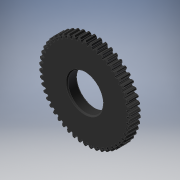
# Autodesk Inventor part: GEFHBS0.5-50-3-10-W0_b
Saved by Autodesk Inventor 2019 (Build 230136000, 136)
## iProperties
Created: 2022-10-16
Part Number: GEFHBS0.5-50-3-10-W0_b
Material: Generic
Catalog Web Link: www.cadenas.de
Description: GEFHB, GEFHBB, GEFHBG, GEFHBS, GEFB, GEFBB, GEFBG, GEFBS, GEFKB, GEFKBB, GEFKBG, GEFKBS_body-Spur Gears - Tooth Width, Hub Dimensions Configurable - Pressure Angle 20degree Module 0.5 / 0.8 / 1.0 / 1.5 / 2.0 / 2.5 / 3.0
Vendor: MISUMI
Document SubType Name: Modeling
Designer: psAdmin
Manufacturer: MISUMI
Mass: 1.22085 g
Surface Area: 13.5083 cm^2
Volume: 1.22085 cm^3
Density: 1 g/cm^3
Appearance: PSOLRGB-175-175-175
Category: PARTsolutions
Company: MISUMI
Title: GEFHBS0.5-50-3-10-W0
Author: Cadenas PARTsolutions
Comments: Spur Gears - Tooth Width, Hub Dimensions Configurable - Pressure Angle 20degree Module 0.5 / 0.8 / 1.0 / 1.5 / 2.0 / 2.5 / 3.0
PSOL_IDENT_0: {$CADENAS_DATA/23d-libs/misumi/metric/54_spur_gears/gefhb/gefhb.prj},485 {VTYP=3D},{NB=GEFHBS0.5-50-
PSOL_IDENT_1: 3-10-W0_b},{LINA=GEFHBS0.5-50-3-10-W0},{NN=GEFHB, GEFHBB, GEFHBG, GEFHBS, GEFB, GEFBB, GEFBG, GEFBS,
PSOL_IDENT_2: GEFKB, GEFKBB, GEFKBG, GEFKBS_body},{DATE=07.06.2021 01:25:58},{GEOMDATE=09.07.2020 06:30:05},{VERS
PSOL_IDENT_3: ION=},{LINEID=10},{WBVAR=SHS,MAT,ST,NT,B,PS,ALT2,TPC,W,H,ALT1,ALT11,ALT4,Z,J,ALT5,Q,R,S,T,ALT9,SRG,A
PSOL_IDENT_4: LT6,LFC,LTC,MALT6,ALT7,KFC,KTC,K,ALT3,DIRALT3,QFC,QTC,MALT3,ALT8,DIRALT8,ZFC,ZTC,U},{WBNUMERIC=NT,B,
PSOL_IDENT_5: W,H,Z,J,Q,R,S,T,SRG,LFC,LTC,KFC,KTC,K,QFC,QTC,ZFC,ZTC,U}  {NB=GEFHBS0.5-50-3-10-W0_b},{LINA=GEFHBS0.
PSOL_IDENT_6: 5-50-3-10-W0},{KT=DUMMY},{PN=GEFHBS0.5-50-3-10-W0},{TYPE=GEFHBS},{SHS=RH},{SHSALG= 'RH','Round Hole'
PSOL_IDENT_7: ,'RHT','Round Hole+Tap' },{MAT=SUS304},{MATALG='S45C', 'S45C Equivalent', 'SUS304', 'SUS304'},{ST=},
PSOL_IDENT_8: {STALG= '','-'},{MOD=0.5},{MOD1=0.5},{AC=N/A},{NT=50},{NTALG=20,24,25,26,30,32,36,40,48,50},{NTALG1=
PSOL_IDENT_9: 20,24,25,26,30,32,36,40,48,50},{NTALG2=0},{NTALG3=24,25,26,30,32,36,40,48,50},{B=3},{BA=[2:5/1]},{PS=
PSOL_IDENT_10: 10},{PALG='3','3','4','4','5','5','6','6','6.35','6.35','7','7','8','8','9','9','10','10','11','11','
PSOL_IDENT_11: 12','12'},{PA1='3','3','4','4','5','5','6','6','6.35','6.35','7','7','8','8','9','9','10','10','11','
PSOL_IDENT_12: 11','12','12'},{PA2='0'},{PA3='3','3','4','4','5','5','6','6','6.35','6.35','7','7','8','8','9','9','
PSOL_IDENT_13: 10','10','11','11','12','12'},{P=10.00},{P2=10},{ALT2=},{ALT2ALG='','N/A'},{TPC=N/A},{TPCALG= 'N/A'
PSOL_IDENT_14: },{ALT2PN=},{W=0},{WA=[0:10/1]},{WMA=0},{H=0},{HA=0},{HMIN=12.0},{HMAX=21},{HPN=},{DD=25.0},{D=26.0}
PSOL_IDENT_15: ,{G=23.75},{M=-},{ML=0},{ACSS=-},{BB=0},{TT=0.0},{L=3},{LL2=0},{ALT1=},{ALT1ALG= '','N/A' },{ALT1PN=
PSOL_IDENT_16: },{KC=0.000},{ALT11=},{ALT11ALG= '','N/A' },{ALT11PN=},{DEG=0},{ALT4=},{ALT4ALG='','Not applicable'}
PSOL_IDENT_17: ,{ALT4PN=},{ALT41=0},{ALT42=0},{Z=0},{ZMINL=12},{ZMAXL=19},{ZMINR=12},{ZMAXR=19},{ZALG=0},{ZPN=},{J=
PSOL_IDENT_18: 0.0},{JALG=0},{JMIN=2},{JMAX=0},{JPN=},{ALT5=},{ALT5ALG= '','Not applicable' },{ALT5PN=},{Q=0},{QALG=
PSOL_IDENT_19: 0},{QMIN=12},{QMAX=19},{QPN=},{R=0},{RALG=0},{RMIN=12},{RMAX=19},{RPN=},{S=0},{SALG=0},{SMIN=3},{SMA
PSOL_IDENT_20: X=-3},{SPN=},{T=0},{TALG=0},{TMIN=3},{TMAX=0},{TPN=},{ALT9=},{ALT9ALG= '','Not applicable' },{SRG=0.
PSOL_IDENT_21: 0},{SRGALG=0},{SRGMIN=3.500},{SRGMINALG=3.500},{SRGMAX=0.000},{SRGMAXALG=0.000},{DD2=0.0},{MM=0.00},
PSOL_IDENT_22: {NN=0.00},{DD2ALG=0.000},{MMALG=0.000},{NNALG=0.000},{ALT9PN=},{ALT6=},{ALT6ALG= '','Not applicable'
PSOL_IDENT_23: },{ALT6PN=},{LFC=0},{LFCALG=0},{LTC=0},{LTCALG=0},{LPCDMIN=18},{LPCDMAX=16},{MALT6=N/A},{MALT6ALG= '
PSOL_IDENT_24: N/A' },{C=0.0},{ALT7=},{ALT7ALG= '','Not applicable' },{ALT7PN=},{KFC=0},{KFCALG=[0]},{KTC=0},{KTCAL
PSOL_IDENT_25: G=[0]},{KPCDMIN1=17},{KPCDMAX1=-7},{KPCDMIN2=7},{KPCDMAX2=16},{K=0.0},{KALG=[0]},{KALT7L=3},{TIF=1},
PSOL_IDENT_26: {KPCD=0},{SCREW=0},{SCREWL=6},{PLANE=5},{PLANE1=5},{ALT3=},{ALT3ALG= '','Not applicable' },{ALT3PN=}
PSOL_IDENT_27: ,{DIRALT3=},{DIRALT3ALG= '','N/A' },{QFC=0},{QFCALG=[0]},{QTC=0},{QTCALG=[0]},{QPCDMIN1=17},{QPCDMAX
PSOL_IDENT_28: 1=-7},{QPCDMIN2=7},{QPCDMAX2=16},{QPCD=0},{CIFMALT3=3},{MALT3=N/A},{MALT3ALG= 'N/A' },{MALT3L=0},{MS
PSOL_IDENT_29: 1=3},{MMAX=1},{MIN=2},{MAX=2},{PITCH=0},{ALT8=},{ALT8ALG= '','Not applicable' },{ALT8PN=},{DIRALT8=}
PSOL_IDENT_30: ,{DIRALT8ALG= '','N/A' },{ZFC=0},{ZFCALG=[0]},{ZTC=0},{ZTCALG=[0]},{ZPCDMIN1=20},{ZPCDMIN2=11},{ZPCD
PSOL_IDENT_31: MAX1=-10},{ZPCDMAX2=13},{ZPCD=0},{U=0},{UALG=[0]},{UMAX=0},{UMAX1=0},{UMAX2=0},{UMIN=3},{U1=0.0},{U2=
PSOL_IDENT_32: 0.0},{F=0.0},{LL13D=0},{LL23D=0},{PZQRDD2=10},{LBS=3},{PCD=0},{SHN=0},{SHDEG1=0},{SHDEG2=0},{ALT3LBS=
PSOL_IDENT_33: 2.5},{D1=1.8},{D2=3.6},{D3=20},{D4=0.05},{D5=4.166667},{D6=3.846154},{D7=0.425},{D8=0.25},{D9=0.4133
PSOL_IDENT_34: 12},{S1=15},{S2=0.5}
NB: GEFHBS0.5-50-3-10-W0_b
NN: 0
NT: 50
NBSYN: $PN._b
LINA: GEFHBS0.5-50-3-10-W0
CATALOG: Misumi
PN: GEFHBS0.5-50-3-10-W0
SHS: Round Hole
MAT: SUS304
ST: -
MOD: 0.5
B: 3
PS: 10
ALT2: N/A
TPC: N/A
W: 0
H: 0
DD: 25
D: 26
G: 23.75
M: -
ACSS: -
ALT1: N/A
ALT11: N/A
ALT4: Not applicable
Z: 0
J: 0
ALT5: Not applicable
Q: 0
R: 0
S: 0
T: 0
ALT9: Not applicable
SRG: 0
DD2: 0
MM: 0
ALT6: Not applicable
LFC: 0
LTC: 0
MALT6: N/A
C: 0
ALT7: Not applicable
KFC: 0
KTC: 0
K: 0
ALT3: Not applicable
DIRALT3: N/A
QFC: 0
QTC: 0
MALT3: N/A
ALT8: Not applicable
DIRALT8: N/A
ZFC: 0
ZTC: 0
U: 0
U1: 0
U2: 0
F: 0
SUPPLIER: MISUMI
ARTICLENO: GEFHBS0.5-50-3-10-W0_b
BOMINFO: GEFHBS0.5-50-3-10-W0
CREATOR: CADENAS GmbH
Autodesk Inventor part; units mm, degrees
(part 1 of 2)
sketch "_____14" plane through (0, 0, 0) normal (1, 0, 0) x (0, 0, -1)
  line L0 (0, 0) -> (-3, 0)
  line L1 (-3, 0) -> (-3, 12.5)
  line L2 (-3, 12.5) -> (-2.3301, 15)
  line L3 (-2.3301, 15) -> (-0.6699, 15)
  line L4 (-0.6699, 15) -> (0, 12.5)
  line L5 (0, 12.5) -> (0, 0)
  line L6 (0, 0) -> (-3, 0)
  constraints: 14 end point
revolve "Revolution1" add sketch "_____14" angle 360 about axis through (0, 0, 0) along (0, 0, -1)
sketch "Sketch_3" plane through (0, 0, 0) normal (0, 0, 1) x (1, 0, 0)
  circle A0 centre (0, 0) radius 52
  arc A1 (-12.9833, 0.6584) -> (-12.9575, 0.6121) centre (-12.9334, 0.6559) ccw
  arc A2 (-12.9575, 0.6121) -> (-12.4938, 0.3926) centre (-10.9465, 4.2613) ccw
  arc A3 (-12.4938, 0.3926) -> (-12.425, 0.3718) centre (-12.3403, 0.7764) ccw
  arc A4 (-12.0493, 0.2732) -> (-12.425, 0.3718) centre (-13.2129, -3.3927) ccw
  arc A5 (-11.875, 0.0342) -> (-12.0493, 0.2732) centre (-12.1249, 0.0349) ccw
  arc A6 (-11.875, 0.0342) -> (-11.875, -0.0342) centre (0, 0) ccw
  arc A7 (-12.0493, -0.2732) -> (-11.875, -0.0342) centre (-12.1249, -0.0349) ccw
  arc A8 (-12.425, -0.3718) -> (-12.0493, -0.2732) centre (-13.2129, 3.3927) ccw
  arc A9 (-12.425, -0.3718) -> (-12.4938, -0.3926) centre (-12.3403, -0.7764) ccw
  arc A10 (-12.4938, -0.3926) -> (-12.9575, -0.6121) centre (-10.9465, -4.2613) ccw
  arc A11 (-12.9575, -0.6121) -> (-12.9833, -0.6584) centre (-12.9334, -0.6559) ccw
  arc A12 (-12.9833, -0.6584) -> (-12.9635, -0.974) centre (0, 0) ccw
  arc A13 (-12.9635, -0.974) -> (-12.9321, -1.0167) centre (-12.9136, -0.9703) ccw
  arc A14 (-12.9321, -1.0167) -> (-12.4445, -1.1764) centre (-11.3942, 2.8558) ccw
  arc A15 (-12.4445, -1.1764) -> (-12.3736, -1.1884) centre (-12.3403, -0.7764) ccw
  arc A16 (-11.9885, -1.2392) -> (-12.3736, -1.1884) centre (-12.6835, -5.022) ccw
  arc A17 (-11.7856, -1.4544) -> (-11.9885, -1.2392) centre (-12.0337, -1.485) ccw
  arc A18 (-11.7856, -1.4544) -> (-11.777, -1.5222) centre (0, 0) ccw
  arc A19 (-11.9201, -1.7812) -> (-11.777, -1.5222) centre (-12.025, -1.5543) ccw
  arc A20 (-12.2804, -1.9262) -> (-11.9201, -1.7812) centre (-13.534, 1.71) ccw
  arc A21 (-12.2804, -1.9262) -> (-12.3461, -1.9554) centre (-12.1457, -2.3169) ccw
  arc A22 (-12.3461, -1.9554) -> (-12.7786, -2.2313) centre (-10.3261, -5.5997) ccw
  arc A23 (-12.7786, -2.2313) -> (-12.7984, -2.2805) centre (-12.7492, -2.2717) ccw
  arc A24 (-12.7984, -2.2805) -> (-12.7392, -2.5911) centre (0, 0) ccw
  arc A25 (-12.7392, -2.5911) -> (-12.7027, -2.6295) centre (-12.6902, -2.5811) ccw
  arc A26 (-12.7027, -2.6295) -> (-12.199, -2.7268) centre (-11.6623, 1.4052) ccw
  arc A27 (-12.199, -2.7268) -> (-12.1271, -2.7298) centre (-12.1457, -2.3169) ccw
  arc A28 (-11.7387, -2.732) -> (-12.1271, -2.7298) centre (-11.9541, -6.5721) ccw
  arc A29 (-11.5104, -2.9201) -> (-11.7387, -2.732) centre (-11.7527, -2.9816) ccw
  arc A30 (-11.5104, -2.9201) -> (-11.4934, -2.9863) centre (0, 0) ccw
  arc A31 (-11.6028, -3.2611) -> (-11.4934, -2.9863) centre (-11.7353, -3.0491) ccw
  arc A32 (-11.9422, -3.4501) -> (-11.6028, -3.2611) centre (-13.6416, 0.0002) ccw
  arc A33 (-11.9422, -3.4501) -> (-12.0037, -3.4874) centre (-11.7596, -3.8209) ccw
  arc A34 (-12.0037, -3.4874) -> (-12.3982, -3.8153) centre (-9.5428, -6.8497) ccw
  arc A35 (-12.3982, -3.8153) -> (-12.4117, -3.8666) centre (-12.3639, -3.8517) ccw
  arc A36 (-12.4117, -3.8666) -> (-12.314, -4.1673) centre (0, 0) ccw
  arc A37 (-12.314, -4.1673) -> (-12.2729, -4.2009) centre (-12.2666, -4.1513) ccw
  arc A38 (-12.2729, -4.2009) -> (-11.761, -4.2342) centre (-11.7465, -0.0676) ccw
  arc A39 (-11.761, -4.2342) -> (-11.6894, -4.2282) centre (-11.7596, -3.8209) ccw
  arc A40 (-11.3037, -4.1817) -> (-11.6894, -4.2282) centre (-11.0361, -8.0185) ccw
  arc A41 (-11.0536, -4.3397) -> (-11.3037, -4.1817) centre (-11.2863, -4.4311) ccw
  arc A42 (-11.0536, -4.3397) -> (-11.0285, -4.4032) centre (0, 0) ccw
  arc A43 (-11.1026, -4.6896) -> (-11.0285, -4.4032) centre (-11.2607, -4.4959) ccw
  arc A44 (-11.4156, -4.9197) -> (-11.1026, -4.6896) centre (-13.534, -1.7095) ccw
  arc A45 (-11.4156, -4.9197) -> (-11.4719, -4.9643) centre (-11.188, -5.2646) ccw
  arc A46 (-11.4719, -4.9643) -> (-11.8223, -5.3391) centre (-8.6091, -7.9917) ccw
  arc A47 (-11.8223, -5.3391) -> (-11.8292, -5.3917) centre (-11.7837, -5.3709) ccw
  arc A48 (-11.8292, -5.3917) -> (-11.6946, -5.6778) centre (0, 0) ccw
  arc A49 (-11.6946, -5.6778) -> (-11.6496, -5.7059) centre (-11.6496, -5.6559) ccw
  arc A50 (-11.6496, -5.7059) -> (-11.1376, -5.6749) centre (-11.6454, -1.5393) ccw
  arc A51 (-11.1376, -5.6749) -> (-11.0673, -5.6599) centre (-11.1879, -5.2647) ccw
  arc A52 (-10.6905, -5.5654) -> (-11.0673, -5.6599) centre (-9.9441, -9.3385) ccw
  arc A53 (-10.4226, -5.6909) -> (-10.6905, -5.5654) centre (-10.642, -5.8107) ccw
  arc A54 (-10.4226, -5.6909) -> (-10.3896, -5.7507) centre (0, 0) ccw
  arc A55 (-10.4273, -6.0442) -> (-10.3896, -5.7507) centre (-10.6084, -5.8718) ccw
  arc A56 (-10.709, -6.3116) -> (-10.4273, -6.0442) centre (-13.213, -3.3923) ccw
  arc A57 (-10.709, -6.3116) -> (-10.7593, -6.363) centre (-10.4399, -6.6254) ccw
  arc A58 (-10.7593, -6.363) -> (-11.0599, -6.7787) centre (-7.5396, -9.0077) ccw
  arc A59 (-11.0599, -6.7787) -> (-11.0602, -6.8317) centre (-11.0176, -6.8055) ccw
  arc A60 (-11.0602, -6.8317) -> (-10.8907, -7.0987) centre (0, 0) ccw
  arc A61 (-10.8907, -7.0987) -> (-10.8426, -7.121) centre (-10.8488, -7.0714) ccw
  arc A62 (-10.8426, -7.121) -> (-10.3385, -7.026) centre (-11.3606, -2.9867) ccw
  arc A63 (-10.3385, -7.026) -> (-10.2706, -7.0024) centre (-10.4399, -6.6254) ccw
  arc A64 (-9.9087, -6.8614) -> (-10.2706, -7.0024) centre (-8.6953, -10.5111) ccw
  arc A65 (-9.6271, -6.9523) -> (-9.9087, -6.8614) centre (-9.8298, -7.0986) ccw
  arc A66 (-9.6271, -6.9523) -> (-9.587, -7.0076) centre (0, 0) ccw
  arc A67 (-9.5875, -7.3034) -> (-9.587, -7.0076) centre (-9.7888, -7.1551) ccw
  arc A68 (-9.8335, -7.6041) -> (-9.5875, -7.3034) centre (-12.6837, -5.0216) ccw
  arc A69 (-9.8335, -7.6041) -> (-9.8769, -7.6613) centre (-9.5272, -7.8816) ccw
  arc A70 (-9.8769, -7.6613) -> (-10.1231, -8.1114) centre (-6.3511, -9.8817) ccw
  arc A71 (-10.1231, -8.1114) -> (-10.1167, -8.1641) centre (-10.0778, -8.1327) ccw
  arc A72 (-10.1167, -8.1641) -> (-9.9152, -8.4077) centre (0, 0) ccw
  arc A73 (-9.9152, -8.4077) -> (-9.8646, -8.4238) centre (-9.877, -8.3754) ccw
  arc A74 (-9.8646, -8.4238) -> (-9.3764, -8.2664) centre (-10.8967, -4.387) ccw
  arc A75 (-9.3764, -8.2664) -> (-9.312, -8.2344) centre (-9.5272, -7.8816) ccw
  arc A76 (-8.9706, -8.0492) -> (-9.312, -8.2344) centre (-7.3093, -11.5181) ccw
  arc A77 (-8.6799, -8.1041) -> (-8.9706, -8.0492) centre (-8.8626, -8.2747) ccw
  arc A78 (-8.6799, -8.1041) -> (-8.6331, -8.1539) centre (0, 0) ccw
  arc A79 (-8.5966, -8.4475) -> (-8.6331, -8.1539) centre (-8.8148, -8.3255) ccw
  arc A80 (-8.8029, -8.7766) -> (-8.5966, -8.4475) centre (-11.9543, -6.5717) ccw
  arc A81 (-8.8029, -8.7766) -> (-8.8388, -8.8388) centre (-8.4642, -9.0135) ccw
  arc A82 (-8.8388, -8.8388) -> (-9.0266, -9.3162) centre (-5.0626, -10.5997) ccw
  arc A83 (-9.0266, -9.3162) -> (-9.0137, -9.3677) centre (-8.979, -9.3316) ccw
  arc A84 (-9.0137, -9.3677) -> (-8.7832, -9.5841) centre (0, 0) ccw
  arc A85 (-8.7832, -9.5841) -> (-8.7311, -9.5938) centre (-8.7494, -9.5473) ccw
  arc A86 (-8.7311, -9.5938) -> (-8.2664, -9.3764) centre (-10.2609, -5.7181) ccw
  arc A87 (-8.2664, -9.3764) -> (-8.2065, -9.3366) centre (-8.4642, -9.0135) ccw
  arc A88 (-7.891, -9.11) -> (-8.2065, -9.3366) centre (-5.8081, -12.3433) ccw
  arc A89 (-7.5957, -9.128) -> (-7.891, -9.11) centre (-7.7556, -9.3202) ccw
  arc A90 (-7.5957, -9.128) -> (-7.5431, -9.1716) centre (0, 0) ccw
  arc A91 (-7.47, -9.4583) -> (-7.5431, -9.1716) centre (-7.7019, -9.3647) ccw
  arc A92 (-7.6335, -9.8107) -> (-7.47, -9.4583) centre (-11.0364, -8.0181) ccw
  arc A93 (-7.6335, -9.8107) -> (-7.6613, -9.8769) centre (-7.2678, -10.0033) ccw
  arc A94 (-7.6613, -9.8769) -> (-7.7878, -10.3741) centre (-3.6941, -11.1507) ccw
  arc A95 (-7.7878, -10.3741) -> (-7.7685, -10.4235) centre (-7.7387, -10.3834) ccw
  arc A96 (-7.7685, -10.4235) -> (-7.5127, -10.6094) centre (0, 0) ccw
  arc A97 (-7.5127, -10.6094) -> (-7.4598, -10.6124) centre (-7.4838, -10.5686) ccw
  arc A98 (-7.4598, -10.6124) -> (-7.026, -10.3385) centre (-9.4634, -6.9591) ccw
  arc A99 (-7.026, -10.3385) -> (-6.9716, -10.2915) centre (-7.2678, -10.0033) ccw
  arc A100 (-6.687, -10.0272) -> (-6.9716, -10.2915) centre (-4.2153, -12.974) ccw
  arc A101 (-6.3918, -10.008) -> (-6.687, -10.0272) centre (-6.5263, -10.2187) ccw
  arc A102 (-6.3918, -10.008) -> (-6.3341, -10.0447) centre (0, 0) ccw
  arc A103 (-6.2257, -10.3199) -> (-6.3341, -10.0447) centre (-6.4674, -10.2561) ccw
  arc A104 (-6.3437, -10.69) -> (-6.2257, -10.3199) centre (-9.9444, -9.3381) ccw
  arc A105 (-6.3437, -10.69) -> (-6.363, -10.7593) centre (-5.9568, -10.8353) ccw
  arc A106 (-6.363, -10.7593) -> (-6.4262, -11.2684) centre (-2.2675, -11.5257) ccw
  arc A107 (-6.4262, -11.2684) -> (-6.4009, -11.315) centre (-6.3763, -11.2715) ccw
  arc A108 (-6.4009, -11.315) -> (-6.1238, -11.4673) centre (0, 0) ccw
  arc A109 (-6.1238, -11.4673) -> (-6.0709, -11.4637) centre (-6.1002, -11.4232) ccw
  arc A110 (-6.0709, -11.4637) -> (-5.6749, -11.1376) centre (-8.5165, -8.0903) ccw
  arc A111 (-5.6749, -11.1376) -> (-5.6268, -11.0842) centre (-5.9568, -10.8353) ccw
  arc A112 (-5.3775, -10.7862) -> (-5.6268, -11.0842) centre (-2.5559, -13.4) ccw
  arc A113 (-5.087, -10.7302) -> (-5.3775, -10.7862) centre (-5.1941, -10.9561) ccw
  arc A114 (-5.087, -10.7302) -> (-5.0252, -10.7593) centre (0, 0) ccw
  arc A115 (-4.8832, -11.0189) -> (-5.0252, -10.7593) centre (-5.131, -10.9858) ccw
  arc A116 (-4.9539, -11.4008) -> (-4.8832, -11.0189) centre (-8.6956, -10.5108) ccw
  arc A117 (-4.9539, -11.4008) -> (-4.9643, -11.4719) centre (-4.5518, -11.4964) ccw
  arc A118 (-4.9643, -11.4719) -> (-4.9632, -11.9849) centre (-0.805, -11.719) ccw
  arc A119 (-4.9632, -11.9849) -> (-4.9323, -12.028) centre (-4.9133, -11.9817) ccw
  arc A120 (-4.9323, -12.028) -> (-4.6383, -12.1444) centre (0, 0) ccw
  arc A121 (-4.6383, -12.1444) -> (-4.5862, -12.1342) centre (-4.6204, -12.0977) ccw
  arc A122 (-4.5862, -12.1342) -> (-4.2342, -11.761) centre (-7.4354, -9.0939) ccw
  arc A123 (-4.2342, -11.761) -> (-4.1932, -11.702) centre (-4.5518, -11.4964) ccw
  arc A124 (-3.9832, -11.3752) -> (-4.1932, -11.702) centre (-0.8563, -13.6147) ccw
  arc A125 (-3.7021, -11.2832) -> (-3.9832, -11.3752) centre (-3.78, -11.5207) ccw
  arc A126 (-3.7021, -11.2832) -> (-3.6371, -11.3043) centre (0, 0) ccw
  arc A127 (-3.4636, -11.544) -> (-3.6371, -11.3043) centre (-3.7136, -11.5423) ccw
  arc A128 (-3.4859, -11.9318) -> (-3.4636, -11.544) centre (-7.3097, -11.5178) ccw
  arc A129 (-3.4859, -11.9318) -> (-3.4874, -12.0037) centre (-3.075, -11.9763) ccw
  arc A130 (-3.4874, -12.0037) -> (-3.4219, -12.5125) centre (0.6701, -11.7275) ccw
  arc A131 (-3.4219, -12.5125) -> (-3.3859, -12.5513) centre (-3.3728, -12.5031) ccw
  arc A132 (-3.3859, -12.5513) -> (-3.0796, -12.63) centre (0, 0) ccw
  arc A133 (-3.0796, -12.63) -> (-3.0293, -12.6133) centre (-3.0678, -12.5814) ccw
  arc A134 (-3.0293, -12.6133) -> (-2.7268, -12.199) centre (-6.237, -9.9541) ccw
  arc A135 (-2.7268, -12.199) -> (-2.6935, -12.1353) centre (-3.075, -11.9763) ccw
  arc A136 (-2.5261, -11.7847) -> (-2.6935, -12.1353) centre (0.8568, -13.6146) ccw
  arc A137 (-2.2587, -11.6582) -> (-2.5261, -11.7847) centre (-2.3063, -11.9036) ccw
  arc A138 (-2.2587, -11.6582) -> (-2.1916, -11.671) centre (0, 0) ccw
  arc A139 (-1.9895, -11.8871) -> (-2.1916, -11.671) centre (-2.2377, -11.9167) ccw
  arc A140 (-1.963, -12.2746) -> (-1.9895, -11.8871) centre (-5.8085, -12.3431) ccw
  arc A141 (-1.963, -12.2746) -> (-1.9554, -12.3461) centre (-1.5497, -12.2672) ccw
  arc A142 (-1.9554, -12.3461) -> (-1.8267, -12.8427) centre (2.1347, -11.5511) ccw
  arc A143 (-1.8267, -12.8427) -> (-1.7861, -12.8767) centre (-1.7792, -12.8272) ccw
  arc A144 (-1.7861, -12.8767) -> (-1.4724, -12.9164) centre (0, 0) ccw
  arc A145 (-1.4724, -12.9164) -> (-1.4245, -12.8935) centre (-1.4667, -12.8667) ccw
  arc A146 (-1.4245, -12.8935) -> (-1.1764, -12.4445) centre (-4.9403, -10.6573) ccw
  arc A147 (-1.1764, -12.4445) -> (-1.1513, -12.3771) centre (-1.5497, -12.2672) ccw
  arc A148 (-1.0292, -12.0084) -> (-1.1513, -12.3771) centre (2.5564, -13.3999) ccw
  arc A149 (-0.7797, -11.8494) -> (-1.0292, -12.0084) centre (-0.7961, -12.0988) ccw
  arc A150 (-0.7797, -11.8494) -> (-0.7115, -11.8537) centre (0, 0) ccw
  arc A151 (-0.484, -12.0427) -> (-0.7115, -11.8537) centre (-0.7265, -12.1032) ccw
  arc A152 (-0.4091, -12.4238) -> (-0.484, -12.0427) centre (-4.2157, -12.9738) ccw
  arc A153 (-0.4091, -12.4238) -> (-0.3926, -12.4938) centre (0, -12.3647) ccw
  arc A154 (-0.3926, -12.4938) -> (-0.2027, -12.9704) centre (3.5656, -11.1924) ccw
  arc A155 (-0.2027, -12.9704) -> (-0.1581, -12.999) centre (-0.1575, -12.949) ccw
  arc A156 (-0.1581, -12.999) -> (0.1581, -12.999) centre (0, 0) ccw
  arc A157 (0.1581, -12.999) -> (0.2027, -12.9704) centre (0.1575, -12.949) ccw
  arc A158 (0.2027, -12.9704) -> (0.3926, -12.4938) centre (-3.5656, -11.1924) ccw
  arc A159 (0.3926, -12.4938) -> (0.4091, -12.4238) centre (0, -12.3647) ccw
  arc A160 (0.484, -12.0427) -> (0.4091, -12.4238) centre (4.2157, -12.9738) ccw
  arc A161 (0.7115, -11.8537) -> (0.484, -12.0427) centre (0.7265, -12.1032) ccw
  arc A162 (0.7115, -11.8537) -> (0.7797, -11.8494) centre (0, 0) ccw
  arc A163 (1.0292, -12.0084) -> (0.7797, -11.8494) centre (0.7961, -12.0988) ccw
  arc A164 (1.1513, -12.3771) -> (1.0292, -12.0084) centre (-2.5564, -13.3999) ccw
  arc A165 (1.1513, -12.3771) -> (1.1764, -12.4445) centre (1.5497, -12.2672) ccw
  arc A166 (1.1764, -12.4445) -> (1.4245, -12.8935) centre (4.9403, -10.6573) ccw
  arc A167 (1.4245, -12.8935) -> (1.4724, -12.9164) centre (1.4667, -12.8667) ccw
  arc A168 (1.4724, -12.9164) -> (1.7861, -12.8767) centre (0, 0) ccw
  arc A169 (1.7861, -12.8767) -> (1.8267, -12.8427) centre (1.7792, -12.8272) ccw
  arc A170 (1.8267, -12.8427) -> (1.9554, -12.3461) centre (-2.1347, -11.5511) ccw
  arc A171 (1.9554, -12.3461) -> (1.963, -12.2746) centre (1.5497, -12.2672) ccw
  arc A172 (1.9895, -11.8871) -> (1.963, -12.2746) centre (5.8085, -12.3431) ccw
  arc A173 (2.1916, -11.671) -> (1.9895, -11.8871) centre (2.2377, -11.9167) ccw
  arc A174 (2.1916, -11.671) -> (2.2587, -11.6582) centre (0, 0) ccw
  arc A175 (2.5261, -11.7847) -> (2.2587, -11.6582) centre (2.3063, -11.9036) ccw
  arc A176 (2.6935, -12.1353) -> (2.5261, -11.7847) centre (-0.8568, -13.6146) ccw
  arc A177 (2.6935, -12.1353) -> (2.7268, -12.199) centre (3.075, -11.9763) ccw
  arc A178 (2.7268, -12.199) -> (3.0293, -12.6133) centre (6.237, -9.9541) ccw
  arc A179 (3.0293, -12.6133) -> (3.0796, -12.63) centre (3.0678, -12.5814) ccw
  arc A180 (3.0796, -12.63) -> (3.3859, -12.5513) centre (0, 0) ccw
  arc A181 (3.3859, -12.5513) -> (3.4219, -12.5125) centre (3.3728, -12.5031) ccw
  arc A182 (3.4219, -12.5125) -> (3.4874, -12.0037) centre (-0.6701, -11.7275) ccw
  arc A183 (3.4874, -12.0037) -> (3.4859, -11.9318) centre (3.075, -11.9763) ccw
  arc A184 (3.4636, -11.544) -> (3.4859, -11.9318) centre (7.3097, -11.5178) ccw
  arc A185 (3.6371, -11.3043) -> (3.4636, -11.544) centre (3.7136, -11.5423) ccw
  arc A186 (3.6371, -11.3043) -> (3.7021, -11.2832) centre (0, 0) ccw
  arc A187 (3.9832, -11.3752) -> (3.7021, -11.2832) centre (3.78, -11.5207) ccw
  arc A188 (4.1932, -11.702) -> (3.9832, -11.3752) centre (0.8563, -13.6147) ccw
  arc A189 (4.1932, -11.702) -> (4.2342, -11.761) centre (4.5518, -11.4964) ccw
  arc A190 (4.2342, -11.761) -> (4.5862, -12.1342) centre (7.4354, -9.0939) ccw
  arc A191 (4.5862, -12.1342) -> (4.6383, -12.1444) centre (4.6204, -12.0977) ccw
  arc A192 (4.6383, -12.1444) -> (4.9323, -12.028) centre (0, 0) ccw
  arc A193 (4.9323, -12.028) -> (4.9632, -11.9849) centre (4.9133, -11.9817) ccw
  arc A194 (4.9632, -11.9849) -> (4.9643, -11.4719) centre (0.805, -11.719) ccw
  arc A195 (4.9643, -11.4719) -> (4.9539, -11.4008) centre (4.5518, -11.4964) ccw
  arc A196 (4.8832, -11.0189) -> (4.9539, -11.4008) centre (8.6956, -10.5108) ccw
  arc A197 (5.0252, -10.7593) -> (4.8832, -11.0189) centre (5.131, -10.9858) ccw
  arc A198 (5.0252, -10.7593) -> (5.087, -10.7302) centre (0, 0) ccw
  arc A199 (5.3775, -10.7862) -> (5.087, -10.7302) centre (5.1941, -10.9561) ccw
  arc A200 (5.6268, -11.0842) -> (5.3775, -10.7862) centre (2.5559, -13.4) ccw
  arc A201 (5.6268, -11.0842) -> (5.6749, -11.1376) centre (5.9568, -10.8353) ccw
  arc A202 (5.6749, -11.1376) -> (6.0709, -11.4637) centre (8.5165, -8.0903) ccw
  arc A203 (6.0709, -11.4637) -> (6.1238, -11.4673) centre (6.1002, -11.4232) ccw
  arc A204 (6.1238, -11.4673) -> (6.4009, -11.315) centre (0, 0) ccw
  arc A205 (6.4009, -11.315) -> (6.4262, -11.2684) centre (6.3763, -11.2715) ccw
  arc A206 (6.4262, -11.2684) -> (6.363, -10.7593) centre (2.2675, -11.5257) ccw
  arc A207 (6.363, -10.7593) -> (6.3437, -10.69) centre (5.9568, -10.8353) ccw
  arc A208 (6.2257, -10.3199) -> (6.3437, -10.69) centre (9.9444, -9.3381) ccw
  arc A209 (6.3341, -10.0447) -> (6.2257, -10.3199) centre (6.4674, -10.2561) ccw
  arc A210 (6.3341, -10.0447) -> (6.3918, -10.008) centre (0, 0) ccw
  arc A211 (6.687, -10.0272) -> (6.3918, -10.008) centre (6.5263, -10.2187) ccw
  arc A212 (6.9716, -10.2915) -> (6.687, -10.0272) centre (4.2153, -12.974) ccw
  arc A213 (6.9716, -10.2915) -> (7.026, -10.3385) centre (7.2678, -10.0033) ccw
  arc A214 (7.026, -10.3385) -> (7.4598, -10.6124) centre (9.4634, -6.9591) ccw
  arc A215 (7.4598, -10.6124) -> (7.5127, -10.6094) centre (7.4838, -10.5686) ccw
  arc A216 (7.5127, -10.6094) -> (7.7685, -10.4235) centre (0, 0) ccw
  arc A217 (7.7685, -10.4235) -> (7.7878, -10.3741) centre (7.7387, -10.3834) ccw
  arc A218 (7.7878, -10.3741) -> (7.6613, -9.8769) centre (3.6941, -11.1507) ccw
  arc A219 (7.6613, -9.8769) -> (7.6335, -9.8107) centre (7.2678, -10.0033) ccw
  arc A220 (7.47, -9.4583) -> (7.6335, -9.8107) centre (11.0364, -8.0181) ccw
  arc A221 (7.5431, -9.1716) -> (7.47, -9.4583) centre (7.7019, -9.3647) ccw
  arc A222 (7.5431, -9.1716) -> (7.5957, -9.128) centre (0, 0) ccw
  arc A223 (7.891, -9.11) -> (7.5957, -9.128) centre (7.7556, -9.3202) ccw
  arc A224 (8.2065, -9.3366) -> (7.891, -9.11) centre (5.8081, -12.3433) ccw
  arc A225 (8.2065, -9.3366) -> (8.2664, -9.3764) centre (8.4642, -9.0135) ccw
  arc A226 (8.2664, -9.3764) -> (8.7311, -9.5938) centre (10.2609, -5.7181) ccw
  arc A227 (8.7311, -9.5938) -> (8.7832, -9.5841) centre (8.7494, -9.5473) ccw
  arc A228 (8.7832, -9.5841) -> (9.0137, -9.3677) centre (0, 0) ccw
  arc A229 (9.0137, -9.3677) -> (9.0266, -9.3162) centre (8.979, -9.3316) ccw
  arc A230 (9.0266, -9.3162) -> (8.8388, -8.8388) centre (5.0626, -10.5997) ccw
  arc A231 (8.8388, -8.8388) -> (8.8029, -8.7766) centre (8.4642, -9.0135) ccw
  arc A232 (8.5966, -8.4475) -> (8.8029, -8.7766) centre (11.9543, -6.5717) ccw
  arc A233 (8.6331, -8.1539) -> (8.5966, -8.4475) centre (8.8148, -8.3255) ccw
  arc A234 (8.6331, -8.1539) -> (8.6799, -8.1041) centre (0, 0) ccw
  arc A235 (8.9706, -8.0492) -> (8.6799, -8.1041) centre (8.8626, -8.2747) ccw
  arc A236 (9.312, -8.2344) -> (8.9706, -8.0492) centre (7.3093, -11.5181) ccw
  arc A237 (9.312, -8.2344) -> (9.3764, -8.2664) centre (9.5272, -7.8816) ccw
  arc A238 (9.3764, -8.2664) -> (9.8646, -8.4238) centre (10.8967, -4.387) ccw
  arc A239 (9.8646, -8.4238) -> (9.9152, -8.4077) centre (9.877, -8.3754) ccw
  arc A240 (9.9152, -8.4077) -> (10.1167, -8.1641) centre (0, 0) ccw
  arc A241 (10.1167, -8.1641) -> (10.1231, -8.1114) centre (10.0778, -8.1327) ccw
  arc A242 (10.1231, -8.1114) -> (9.8769, -7.6613) centre (6.3511, -9.8817) ccw
  arc A243 (9.8769, -7.6613) -> (9.8335, -7.6041) centre (9.5272, -7.8816) ccw
  arc A244 (9.5875, -7.3034) -> (9.8335, -7.6041) centre (12.6837, -5.0216) ccw
  arc A245 (9.587, -7.0076) -> (9.5875, -7.3034) centre (9.7888, -7.1551) ccw
  arc A246 (9.587, -7.0076) -> (9.6271, -6.9523) centre (0, 0) ccw
  arc A247 (9.9087, -6.8614) -> (9.6271, -6.9523) centre (9.8298, -7.0986) ccw
  arc A248 (10.2706, -7.0024) -> (9.9087, -6.8614) centre (8.6953, -10.5111) ccw
  arc A249 (10.2706, -7.0024) -> (10.3385, -7.026) centre (10.4399, -6.6254) ccw
  arc A250 (10.3385, -7.026) -> (10.8426, -7.121) centre (11.3606, -2.9867) ccw
  arc A251 (10.8426, -7.121) -> (10.8907, -7.0987) centre (10.8488, -7.0714) ccw
  arc A252 (10.8907, -7.0987) -> (11.0602, -6.8317) centre (0, 0) ccw
  arc A253 (11.0602, -6.8317) -> (11.0599, -6.7787) centre (11.0176, -6.8055) ccw
  arc A254 (11.0599, -6.7787) -> (10.7593, -6.363) centre (7.5396, -9.0077) ccw
  arc A255 (10.7593, -6.363) -> (10.709, -6.3116) centre (10.4399, -6.6254) ccw
  arc A256 (10.4273, -6.0442) -> (10.709, -6.3116) centre (13.213, -3.3923) ccw
  arc A257 (10.3896, -5.7507) -> (10.4273, -6.0442) centre (10.6084, -5.8718) ccw
  arc A258 (10.3896, -5.7507) -> (10.4226, -5.6909) centre (0, 0) ccw
  arc A259 (10.6905, -5.5654) -> (10.4226, -5.6909) centre (10.642, -5.8107) ccw
  arc A260 (11.0673, -5.6599) -> (10.6905, -5.5654) centre (9.9441, -9.3385) ccw
  arc A261 (11.0673, -5.6599) -> (11.1376, -5.6749) centre (11.1879, -5.2647) ccw
  arc A262 (11.1376, -5.6749) -> (11.6496, -5.7059) centre (11.6454, -1.5393) ccw
  arc A263 (11.6496, -5.7059) -> (11.6946, -5.6778) centre (11.6496, -5.6559) ccw
  arc A264 (11.6946, -5.6778) -> (11.8292, -5.3917) centre (0, 0) ccw
  arc A265 (11.8292, -5.3917) -> (11.8223, -5.3391) centre (11.7837, -5.3709) ccw
  arc A266 (11.8223, -5.3391) -> (11.4719, -4.9643) centre (8.6091, -7.9917) ccw
  arc A267 (11.4719, -4.9643) -> (11.4156, -4.9197) centre (11.188, -5.2646) ccw
  arc A268 (11.1026, -4.6896) -> (11.4156, -4.9197) centre (13.534, -1.7095) ccw
  arc A269 (11.0285, -4.4032) -> (11.1026, -4.6896) centre (11.2607, -4.4959) ccw
  arc A270 (11.0285, -4.4032) -> (11.0536, -4.3397) centre (0, 0) ccw
  arc A271 (11.3037, -4.1817) -> (11.0536, -4.3397) centre (11.2863, -4.4311) ccw
  arc A272 (11.6894, -4.2282) -> (11.3037, -4.1817) centre (11.0361, -8.0185) ccw
  arc A273 (11.6894, -4.2282) -> (11.761, -4.2342) centre (11.7596, -3.8209) ccw
  arc A274 (11.761, -4.2342) -> (12.2729, -4.2009) centre (11.7465, -0.0676) ccw
  arc A275 (12.2729, -4.2009) -> (12.314, -4.1673) centre (12.2666, -4.1513) ccw
  arc A276 (12.314, -4.1673) -> (12.4117, -3.8666) centre (0, 0) ccw
  arc A277 (12.4117, -3.8666) -> (12.3982, -3.8153) centre (12.3639, -3.8517) ccw
  arc A278 (12.3982, -3.8153) -> (12.0037, -3.4874) centre (9.5428, -6.8497) ccw
  arc A279 (12.0037, -3.4874) -> (11.9422, -3.4501) centre (11.7596, -3.8209) ccw
  arc A280 (11.6028, -3.2611) -> (11.9422, -3.4501) centre (13.6416, 0.0002) ccw
  arc A281 (11.4934, -2.9863) -> (11.6028, -3.2611) centre (11.7353, -3.0491) ccw
  arc A282 (11.4934, -2.9863) -> (11.5104, -2.9201) centre (0, 0) ccw
  arc A283 (11.7387, -2.732) -> (11.5104, -2.9201) centre (11.7527, -2.9816) ccw
  arc A284 (12.1271, -2.7298) -> (11.7387, -2.732) centre (11.9541, -6.5721) ccw
  arc A285 (12.1271, -2.7298) -> (12.199, -2.7268) centre (12.1457, -2.3169) ccw
  arc A286 (12.199, -2.7268) -> (12.7027, -2.6295) centre (11.6623, 1.4052) ccw
  arc A287 (12.7027, -2.6295) -> (12.7392, -2.5911) centre (12.6902, -2.5811) ccw
  arc A288 (12.7392, -2.5911) -> (12.7984, -2.2805) centre (0, 0) ccw
  arc A289 (12.7984, -2.2805) -> (12.7786, -2.2313) centre (12.7492, -2.2717) ccw
  arc A290 (12.7786, -2.2313) -> (12.3461, -1.9554) centre (10.3261, -5.5997) ccw
  arc A291 (12.3461, -1.9554) -> (12.2804, -1.9262) centre (12.1457, -2.3169) ccw
  arc A292 (11.9201, -1.7812) -> (12.2804, -1.9262) centre (13.534, 1.71) ccw
  arc A293 (11.777, -1.5222) -> (11.9201, -1.7812) centre (12.025, -1.5543) ccw
  arc A294 (11.777, -1.5222) -> (11.7856, -1.4544) centre (0, 0) ccw
  arc A295 (11.9885, -1.2392) -> (11.7856, -1.4544) centre (12.0337, -1.485) ccw
  arc A296 (12.3736, -1.1884) -> (11.9885, -1.2392) centre (12.6835, -5.022) ccw
  arc A297 (12.3736, -1.1884) -> (12.4445, -1.1764) centre (12.3403, -0.7764) ccw
  arc A298 (12.4445, -1.1764) -> (12.9321, -1.0167) centre (11.3942, 2.8558) ccw
  arc A299 (12.9321, -1.0167) -> (12.9635, -0.974) centre (12.9136, -0.9703) ccw
  arc A300 (12.9635, -0.974) -> (12.9833, -0.6584) centre (0, 0) ccw
  arc A301 (12.9833, -0.6584) -> (12.9575, -0.6121) centre (12.9334, -0.6559) ccw
  arc A302 (12.9575, -0.6121) -> (12.4938, -0.3926) centre (10.9465, -4.2613) ccw
  arc A303 (12.4938, -0.3926) -> (12.425, -0.3718) centre (12.3403, -0.7764) ccw
  arc A304 (12.0493, -0.2732) -> (12.425, -0.3718) centre (13.2129, 3.3927) ccw
  arc A305 (11.875, -0.0342) -> (12.0493, -0.2732) centre (12.1249, -0.0349) ccw
  arc A306 (11.875, -0.0342) -> (11.875, 0.0342) centre (0, 0) ccw
  arc A307 (12.0493, 0.2732) -> (11.875, 0.0342) centre (12.1249, 0.0349) ccw
  arc A308 (12.425, 0.3718) -> (12.0493, 0.2732) centre (13.2129, -3.3927) ccw
  arc A309 (12.425, 0.3718) -> (12.4938, 0.3926) centre (12.3403, 0.7764) ccw
  arc A310 (12.4938, 0.3926) -> (12.9575, 0.6121) centre (10.9465, 4.2613) ccw
  arc A311 (12.9575, 0.6121) -> (12.9833, 0.6584) centre (12.9334, 0.6559) ccw
  arc A312 (12.9833, 0.6584) -> (12.9635, 0.974) centre (0, 0) ccw
  arc A313 (12.9635, 0.974) -> (12.9321, 1.0167) centre (12.9136, 0.9703) ccw
  arc A314 (12.9321, 1.0167) -> (12.4445, 1.1764) centre (11.3942, -2.8558) ccw
  arc A315 (12.4445, 1.1764) -> (12.3736, 1.1884) centre (12.3403, 0.7764) ccw
  arc A316 (11.9885, 1.2392) -> (12.3736, 1.1884) centre (12.6835, 5.022) ccw
  arc A317 (11.7856, 1.4544) -> (11.9885, 1.2392) centre (12.0337, 1.485) ccw
  arc A318 (11.7856, 1.4544) -> (11.777, 1.5222) centre (0, 0) ccw
  arc A319 (11.9201, 1.7812) -> (11.777, 1.5222) centre (12.025, 1.5543) ccw
  arc A320 (12.2804, 1.9262) -> (11.9201, 1.7812) centre (13.534, -1.71) ccw
  arc A321 (12.2804, 1.9262) -> (12.3461, 1.9554) centre (12.1457, 2.3169) ccw
  arc A322 (12.3461, 1.9554) -> (12.7786, 2.2313) centre (10.3261, 5.5997) ccw
  arc A323 (12.7786, 2.2313) -> (12.7984, 2.2805) centre (12.7492, 2.2717) ccw
  arc A324 (12.7984, 2.2805) -> (12.7392, 2.5911) centre (0, 0) ccw
  arc A325 (12.7392, 2.5911) -> (12.7027, 2.6295) centre (12.6902, 2.5811) ccw
  arc A326 (12.7027, 2.6295) -> (12.199, 2.7268) centre (11.6623, -1.4052) ccw
  arc A327 (12.199, 2.7268) -> (12.1271, 2.7298) centre (12.1457, 2.3169) ccw
  arc A328 (11.7387, 2.732) -> (12.1271, 2.7298) centre (11.9541, 6.5721) ccw
  arc A329 (11.5104, 2.9201) -> (11.7387, 2.732) centre (11.7527, 2.9816) ccw
  arc A330 (11.5104, 2.9201) -> (11.4934, 2.9863) centre (0, 0) ccw
  arc A331 (11.6028, 3.2611) -> (11.4934, 2.9863) centre (11.7353, 3.0491) ccw
  arc A332 (11.9422, 3.4501) -> (11.6028, 3.2611) centre (13.6416, -0.0002) ccw
  arc A333 (11.9422, 3.4501) -> (12.0037, 3.4874) centre (11.7596, 3.8209) ccw
  arc A334 (12.0037, 3.4874) -> (12.3982, 3.8153) centre (9.5428, 6.8497) ccw
  arc A335 (12.3982, 3.8153) -> (12.4117, 3.8666) centre (12.3639, 3.8517) ccw
  arc A336 (12.4117, 3.8666) -> (12.314, 4.1673) centre (0, 0) ccw
  arc A337 (12.314, 4.1673) -> (12.2729, 4.2009) centre (12.2666, 4.1513) ccw
  arc A338 (12.2729, 4.2009) -> (11.761, 4.2342) centre (11.7465, 0.0676) ccw
  arc A339 (11.761, 4.2342) -> (11.6894, 4.2282) centre (11.7596, 3.8209) ccw
  arc A340 (11.3037, 4.1817) -> (11.6894, 4.2282) centre (11.0361, 8.0185) ccw
  arc A341 (11.0536, 4.3397) -> (11.3037, 4.1817) centre (11.2863, 4.4311) ccw
  arc A342 (11.0536, 4.3397) -> (11.0285, 4.4032) centre (0, 0) ccw
  arc A343 (11.1026, 4.6896) -> (11.0285, 4.4032) centre (11.2607, 4.4959) ccw
  arc A344 (11.4156, 4.9197) -> (11.1026, 4.6896) centre (13.534, 1.7095) ccw
  arc A345 (11.4156, 4.9197) -> (11.4719, 4.9643) centre (11.188, 5.2646) ccw
  arc A346 (11.4719, 4.9643) -> (11.8223, 5.3391) centre (8.6091, 7.9917) ccw
  arc A347 (11.8223, 5.3391) -> (11.8292, 5.3917) centre (11.7837, 5.3709) ccw
  arc A348 (11.8292, 5.3917) -> (11.6946, 5.6778) centre (0, 0) ccw
  arc A349 (11.6946, 5.6778) -> (11.6496, 5.7059) centre (11.6496, 5.6559) ccw
  arc A350 (11.6496, 5.7059) -> (11.1376, 5.6749) centre (11.6454, 1.5393) ccw
  arc A351 (11.1376, 5.6749) -> (11.0673, 5.6599) centre (11.1879, 5.2647) ccw
  arc A352 (10.6905, 5.5654) -> (11.0673, 5.6599) centre (9.9441, 9.3385) ccw
  arc A353 (10.4226, 5.6909) -> (10.6905, 5.5654) centre (10.642, 5.8107) ccw
  arc A354 (10.4226, 5.6909) -> (10.3896, 5.7507) centre (0, 0) ccw
  arc A355 (10.4273, 6.0442) -> (10.3896, 5.7507) centre (10.6084, 5.8718) ccw
  arc A356 (10.709, 6.3116) -> (10.4273, 6.0442) centre (13.213, 3.3923) ccw
  arc A357 (10.709, 6.3116) -> (10.7593, 6.363) centre (10.4399, 6.6254) ccw
  arc A358 (10.7593, 6.363) -> (11.0599, 6.7787) centre (7.5396, 9.0077) ccw
  arc A359 (11.0599, 6.7787) -> (11.0602, 6.8317) centre (11.0176, 6.8055) ccw
  arc A360 (11.0602, 6.8317) -> (10.8907, 7.0987) centre (0, 0) ccw
  arc A361 (10.8907, 7.0987) -> (10.8426, 7.121) centre (10.8488, 7.0714) ccw
  arc A362 (10.8426, 7.121) -> (10.3385, 7.026) centre (11.3606, 2.9867) ccw
  arc A363 (10.3385, 7.026) -> (10.2706, 7.0024) centre (10.4399, 6.6254) ccw
  arc A364 (9.9087, 6.8614) -> (10.2706, 7.0024) centre (8.6953, 10.5111) ccw
  arc A365 (9.6271, 6.9523) -> (9.9087, 6.8614) centre (9.8298, 7.0986) ccw
  arc A366 (9.6271, 6.9523) -> (9.587, 7.0076) centre (0, 0) ccw
  arc A367 (9.5875, 7.3034) -> (9.587, 7.0076) centre (9.7888, 7.1551) ccw
  arc A368 (9.8335, 7.6041) -> (9.5875, 7.3034) centre (12.6837, 5.0216) ccw
  arc A369 (9.8335, 7.6041) -> (9.8769, 7.6613) centre (9.5272, 7.8816) ccw
  arc A370 (9.8769, 7.6613) -> (10.1231, 8.1114) centre (6.3511, 9.8817) ccw
  arc A371 (10.1231, 8.1114) -> (10.1167, 8.1641) centre (10.0778, 8.1327) ccw
  arc A372 (10.1167, 8.1641) -> (9.9152, 8.4077) centre (0, 0) ccw
  arc A373 (9.9152, 8.4077) -> (9.8646, 8.4238) centre (9.877, 8.3754) ccw
  arc A374 (9.8646, 8.4238) -> (9.3764, 8.2664) centre (10.8967, 4.387) ccw
  arc A375 (9.3764, 8.2664) -> (9.312, 8.2344) centre (9.5272, 7.8816) ccw
  arc A376 (8.9706, 8.0492) -> (9.312, 8.2344) centre (7.3093, 11.5181) ccw
  arc A377 (8.6799, 8.1041) -> (8.9706, 8.0492) centre (8.8626, 8.2747) ccw
  arc A378 (8.6799, 8.1041) -> (8.6331, 8.1539) centre (0, 0) ccw
  arc A379 (8.5966, 8.4475) -> (8.6331, 8.1539) centre (8.8148, 8.3255) ccw
  arc A380 (8.8029, 8.7766) -> (8.5966, 8.4475) centre (11.9543, 6.5717) ccw
  arc A381 (8.8029, 8.7766) -> (8.8388, 8.8388) centre (8.4642, 9.0135) ccw
  arc A382 (8.8388, 8.8388) -> (9.0266, 9.3162) centre (5.0626, 10.5997) ccw
  arc A383 (9.0266, 9.3162) -> (9.0137, 9.3677) centre (8.979, 9.3316) ccw
  arc A384 (9.0137, 9.3677) -> (8.7832, 9.5841) centre (0, 0) ccw
  arc A385 (8.7832, 9.5841) -> (8.7311, 9.5938) centre (8.7494, 9.5473) ccw
  arc A386 (8.7311, 9.5938) -> (8.2664, 9.3764) centre (10.2609, 5.7181) ccw
  arc A387 (8.2664, 9.3764) -> (8.2065, 9.3366) centre (8.4642, 9.0135) ccw
  arc A388 (7.891, 9.11) -> (8.2065, 9.3366) centre (5.8081, 12.3433) ccw
  arc A389 (7.5957, 9.128) -> (7.891, 9.11) centre (7.7556, 9.3202) ccw
  arc A390 (7.5957, 9.128) -> (7.5431, 9.1716) centre (0, 0) ccw
  arc A391 (7.47, 9.4583) -> (7.5431, 9.1716) centre (7.7019, 9.3647) ccw
  arc A392 (7.6335, 9.8107) -> (7.47, 9.4583) centre (11.0364, 8.0181) ccw
  arc A393 (7.6335, 9.8107) -> (7.6613, 9.8769) centre (7.2678, 10.0033) ccw
  arc A394 (7.6613, 9.8769) -> (7.7878, 10.3741) centre (3.6941, 11.1507) ccw
  arc A395 (7.7878, 10.3741) -> (7.7685, 10.4235) centre (7.7387, 10.3834) ccw
  arc A396 (7.7685, 10.4235) -> (7.5127, 10.6094) centre (0, 0) ccw
  arc A397 (7.5127, 10.6094) -> (7.4598, 10.6124) centre (7.4838, 10.5686) ccw
  arc A398 (7.4598, 10.6124) -> (7.026, 10.3385) centre (9.4634, 6.9591) ccw
  arc A399 (7.026, 10.3385) -> (6.9716, 10.2915) centre (7.2678, 10.0033) ccw
  arc A400 (6.687, 10.0272) -> (6.9716, 10.2915) centre (4.2153, 12.974) ccw
  arc A401 (6.3918, 10.008) -> (6.687, 10.0272) centre (6.5263, 10.2187) ccw
  arc A402 (6.3918, 10.008) -> (6.3341, 10.0447) centre (0, 0) ccw
  arc A403 (6.2257, 10.3199) -> (6.3341, 10.0447) centre (6.4674, 10.2561) ccw
  arc A404 (6.3437, 10.69) -> (6.2257, 10.3199) centre (9.9444, 9.3381) ccw
  arc A405 (6.3437, 10.69) -> (6.363, 10.7593) centre (5.9568, 10.8353) ccw
  arc A406 (6.363, 10.7593) -> (6.4262, 11.2684) centre (2.2675, 11.5257) ccw
  arc A407 (6.4262, 11.2684) -> (6.4009, 11.315) centre (6.3763, 11.2715) ccw
  arc A408 (6.4009, 11.315) -> (6.1238, 11.4673) centre (0, 0) ccw
  arc A409 (6.1238, 11.4673) -> (6.0709, 11.4637) centre (6.1002, 11.4232) ccw
  arc A410 (6.0709, 11.4637) -> (5.6749, 11.1376) centre (8.5165, 8.0903) ccw
  arc A411 (5.6749, 11.1376) -> (5.6268, 11.0842) centre (5.9568, 10.8353) ccw
  arc A412 (5.3775, 10.7862) -> (5.6268, 11.0842) centre (2.5559, 13.4) ccw
  arc A413 (5.087, 10.7302) -> (5.3775, 10.7862) centre (5.1941, 10.9561) ccw
  arc A414 (5.087, 10.7302) -> (5.0252, 10.7593) centre (0, 0) ccw
  arc A415 (4.8832, 11.0189) -> (5.0252, 10.7593) centre (5.131, 10.9858) ccw
  arc A416 (4.9539, 11.4008) -> (4.8832, 11.0189) centre (8.6956, 10.5108) ccw
  arc A417 (4.9539, 11.4008) -> (4.9643, 11.4719) centre (4.5518, 11.4964) ccw
  arc A418 (4.9643, 11.4719) -> (4.9632, 11.9849) centre (0.805, 11.719) ccw
  arc A419 (4.9632, 11.9849) -> (4.9323, 12.028) centre (4.9133, 11.9817) ccw
  arc A420 (4.9323, 12.028) -> (4.6383, 12.1444) centre (0, 0) ccw
  arc A421 (4.6383, 12.1444) -> (4.5862, 12.1342) centre (4.6204, 12.0977) ccw
  arc A422 (4.5862, 12.1342) -> (4.2342, 11.761) centre (7.4354, 9.0939) ccw
  arc A423 (4.2342, 11.761) -> (4.1932, 11.702) centre (4.5518, 11.4964) ccw
  arc A424 (3.9832, 11.3752) -> (4.1932, 11.702) centre (0.8563, 13.6147) ccw
  arc A425 (3.7021, 11.2832) -> (3.9832, 11.3752) centre (3.78, 11.5207) ccw
  arc A426 (3.7021, 11.2832) -> (3.6371, 11.3043) centre (0, 0) ccw
  arc A427 (3.4636, 11.544) -> (3.6371, 11.3043) centre (3.7136, 11.5423) ccw
  arc A428 (3.4859, 11.9318) -> (3.4636, 11.544) centre (7.3097, 11.5178) ccw
  arc A429 (3.4859, 11.9318) -> (3.4874, 12.0037) centre (3.075, 11.9763) ccw
  arc A430 (3.4874, 12.0037) -> (3.4219, 12.5125) centre (-0.6701, 11.7275) ccw
  arc A431 (3.4219, 12.5125) -> (3.3859, 12.5513) centre (3.3728, 12.5031) ccw
  arc A432 (3.3859, 12.5513) -> (3.0796, 12.63) centre (0, 0) ccw
  arc A433 (3.0796, 12.63) -> (3.0293, 12.6133) centre (3.0678, 12.5814) ccw
  arc A434 (3.0293, 12.6133) -> (2.7268, 12.199) centre (6.237, 9.9541) ccw
  arc A435 (2.7268, 12.199) -> (2.6935, 12.1353) centre (3.075, 11.9763) ccw
  arc A436 (2.5261, 11.7847) -> (2.6935, 12.1353) centre (-0.8568, 13.6146) ccw
  arc A437 (2.2587, 11.6582) -> (2.5261, 11.7847) centre (2.3063, 11.9036) ccw
  arc A438 (2.2587, 11.6582) -> (2.1916, 11.671) centre (0, 0) ccw
  arc A439 (1.9895, 11.8871) -> (2.1916, 11.671) centre (2.2377, 11.9167) ccw
  arc A440 (1.963, 12.2746) -> (1.9895, 11.8871) centre (5.8085, 12.3431) ccw
  arc A441 (1.963, 12.2746) -> (1.9554, 12.3461) centre (1.5497, 12.2672) ccw
  arc A442 (1.9554, 12.3461) -> (1.8267, 12.8427) centre (-2.1347, 11.5511) ccw
  arc A443 (1.8267, 12.8427) -> (1.7861, 12.8767) centre (1.7792, 12.8272) ccw
  arc A444 (1.7861, 12.8767) -> (1.4724, 12.9164) centre (0, 0) ccw
  arc A445 (1.4724, 12.9164) -> (1.4245, 12.8935) centre (1.4667, 12.8667) ccw
  arc A446 (1.4245, 12.8935) -> (1.1764, 12.4445) centre (4.9403, 10.6573) ccw
  arc A447 (1.1764, 12.4445) -> (1.1513, 12.3771) centre (1.5497, 12.2672) ccw
  arc A448 (1.0292, 12.0084) -> (1.1513, 12.3771) centre (-2.5564, 13.3999) ccw
  arc A449 (0.7797, 11.8494) -> (1.0292, 12.0084) centre (0.7961, 12.0988) ccw
  arc A450 (0.7797, 11.8494) -> (0.7115, 11.8537) centre (0, 0) ccw
  arc A451 (0.484, 12.0427) -> (0.7115, 11.8537) centre (0.7265, 12.1032) ccw
  arc A452 (0.4091, 12.4238) -> (0.484, 12.0427) centre (4.2157, 12.9738) ccw
  arc A453 (0.4091, 12.4238) -> (0.3926, 12.4938) centre (0, 12.3647) ccw
  arc A454 (0.3926, 12.4938) -> (0.2027, 12.9704) centre (-3.5656, 11.1924) ccw
  arc A455 (0.2027, 12.9704) -> (0.1581, 12.999) centre (0.1575, 12.949) ccw
  arc A456 (0.1581, 12.999) -> (-0.1581, 12.999) centre (0, 0) ccw
  arc A457 (-0.1581, 12.999) -> (-0.2027, 12.9704) centre (-0.1575, 12.949) ccw
  arc A458 (-0.2027, 12.9704) -> (-0.3926, 12.4938) centre (3.5656, 11.1924) ccw
  arc A459 (-0.3926, 12.4938) -> (-0.4091, 12.4238) centre (0, 12.3647) ccw
  arc A460 (-0.484, 12.0427) -> (-0.4091, 12.4238) centre (-4.2157, 12.9738) ccw
  arc A461 (-0.7115, 11.8537) -> (-0.484, 12.0427) centre (-0.7265, 12.1032) ccw
  arc A462 (-0.7115, 11.8537) -> (-0.7797, 11.8494) centre (0, 0) ccw
  arc A463 (-1.0292, 12.0084) -> (-0.7797, 11.8494) centre (-0.7961, 12.0988) ccw
  arc A464 (-1.1513, 12.3771) -> (-1.0292, 12.0084) centre (2.5564, 13.3999) ccw
  arc A465 (-1.1513, 12.3771) -> (-1.1764, 12.4445) centre (-1.5497, 12.2672) ccw
  arc A466 (-1.1764, 12.4445) -> (-1.4245, 12.8935) centre (-4.9403, 10.6573) ccw
  arc A467 (-1.4245, 12.8935) -> (-1.4724, 12.9164) centre (-1.4667, 12.8667) ccw
  arc A468 (-1.4724, 12.9164) -> (-1.7861, 12.8767) centre (0, 0) ccw
  arc A469 (-1.7861, 12.8767) -> (-1.8267, 12.8427) centre (-1.7792, 12.8272) ccw
  arc A470 (-1.8267, 12.8427) -> (-1.9554, 12.3461) centre (2.1347, 11.5511) ccw
  arc A471 (-1.9554, 12.3461) -> (-1.963, 12.2746) centre (-1.5497, 12.2672) ccw
  arc A472 (-1.9895, 11.8871) -> (-1.963, 12.2746) centre (-5.8085, 12.3431) ccw
  arc A473 (-2.1916, 11.671) -> (-1.9895, 11.8871) centre (-2.2377, 11.9167) ccw
  arc A474 (-2.1916, 11.671) -> (-2.2587, 11.6582) centre (0, 0) ccw
  arc A475 (-2.5261, 11.7847) -> (-2.2587, 11.6582) centre (-2.3063, 11.9036) ccw
  arc A476 (-2.6935, 12.1353) -> (-2.5261, 11.7847) centre (0.8568, 13.6146) ccw
  arc A477 (-2.6935, 12.1353) -> (-2.7268, 12.199) centre (-3.075, 11.9763) ccw
  arc A478 (-2.7268, 12.199) -> (-3.0293, 12.6133) centre (-6.237, 9.9541) ccw
  arc A479 (-3.0293, 12.6133) -> (-3.0796, 12.63) centre (-3.0678, 12.5814) ccw
  arc A480 (-3.0796, 12.63) -> (-3.3859, 12.5513) centre (0, 0) ccw
  arc A481 (-3.3859, 12.5513) -> (-3.4219, 12.5125) centre (-3.3728, 12.5031) ccw
  arc A482 (-3.4219, 12.5125) -> (-3.4874, 12.0037) centre (0.6701, 11.7275) ccw
  arc A483 (-3.4874, 12.0037) -> (-3.4859, 11.9318) centre (-3.075, 11.9763) ccw
  arc A484 (-3.4636, 11.544) -> (-3.4859, 11.9318) centre (-7.3097, 11.5178) ccw
  arc A485 (-3.6371, 11.3043) -> (-3.4636, 11.544) centre (-3.7136, 11.5423) ccw
  arc A486 (-3.6371, 11.3043) -> (-3.7021, 11.2832) centre (0, 0) ccw
  arc A487 (-3.9832, 11.3752) -> (-3.7021, 11.2832) centre (-3.78, 11.5207) ccw
  arc A488 (-4.1932, 11.702) -> (-3.9832, 11.3752) centre (-0.8563, 13.6147) ccw
  arc A489 (-4.1932, 11.702) -> (-4.2342, 11.761) centre (-4.5518, 11.4964) ccw
  arc A490 (-4.2342, 11.761) -> (-4.5862, 12.1342) centre (-7.4354, 9.0939) ccw
  arc A491 (-4.5862, 12.1342) -> (-4.6383, 12.1444) centre (-4.6204, 12.0977) ccw
  arc A492 (-4.6383, 12.1444) -> (-4.9323, 12.028) centre (0, 0) ccw
  arc A493 (-4.9323, 12.028) -> (-4.9632, 11.9849) centre (-4.9133, 11.9817) ccw
  arc A494 (-4.9632, 11.9849) -> (-4.9643, 11.4719) centre (-0.805, 11.719) ccw
  arc A495 (-4.9643, 11.4719) -> (-4.9539, 11.4008) centre (-4.5518, 11.4964) ccw
  arc A496 (-4.8832, 11.0189) -> (-4.9539, 11.4008) centre (-8.6956, 10.5108) ccw
  arc A497 (-5.0252, 10.7593) -> (-4.8832, 11.0189) centre (-5.131, 10.9858) ccw
  arc A498 (-5.0252, 10.7593) -> (-5.087, 10.7302) centre (0, 0) ccw
  arc A499 (-5.3775, 10.7862) -> (-5.087, 10.7302) centre (-5.1941, 10.9561) ccw
  arc A500 (-5.6268, 11.0842) -> (-5.3775, 10.7862) centre (-2.5559, 13.4) ccw
  arc A501 (-5.6268, 11.0842) -> (-5.6749, 11.1376) centre (-5.9568, 10.8353) ccw
  arc A502 (-5.6749, 11.1376) -> (-6.0709, 11.4637) centre (-8.5165, 8.0903) ccw
  arc A503 (-6.0709, 11.4637) -> (-6.1238, 11.4673) centre (-6.1002, 11.4232) ccw
  arc A504 (-6.1238, 11.4673) -> (-6.4009, 11.315) centre (0, 0) ccw
  arc A505 (-6.4009, 11.315) -> (-6.4262, 11.2684) centre (-6.3763, 11.2715) ccw
  arc A506 (-6.4262, 11.2684) -> (-6.363, 10.7593) centre (-2.2675, 11.5257) ccw
  arc A507 (-6.363, 10.7593) -> (-6.3437, 10.69) centre (-5.9568, 10.8353) ccw
  arc A508 (-6.2257, 10.3199) -> (-6.3437, 10.69) centre (-9.9444, 9.3381) ccw
  arc A509 (-6.3341, 10.0447) -> (-6.2257, 10.3199) centre (-6.4674, 10.2561) ccw
  arc A510 (-6.3341, 10.0447) -> (-6.3918, 10.008) centre (0, 0) ccw
  arc A511 (-6.687, 10.0272) -> (-6.3918, 10.008) centre (-6.5263, 10.2187) ccw
  arc A512 (-6.9716, 10.2915) -> (-6.687, 10.0272) centre (-4.2153, 12.974) ccw
  arc A513 (-6.9716, 10.2915) -> (-7.026, 10.3385) centre (-7.2678, 10.0033) ccw
  arc A514 (-7.026, 10.3385) -> (-7.4598, 10.6124) centre (-9.4634, 6.9591) ccw
  arc A515 (-7.4598, 10.6124) -> (-7.5127, 10.6094) centre (-7.4838, 10.5686) ccw
  arc A516 (-7.5127, 10.6094) -> (-7.7685, 10.4235) centre (0, 0) ccw
  arc A517 (-7.7685, 10.4235) -> (-7.7878, 10.3741) centre (-7.7387, 10.3834) ccw
  arc A518 (-7.7878, 10.3741) -> (-7.6613, 9.8769) centre (-3.6941, 11.1507) ccw
  arc A519 (-7.6613, 9.8769) -> (-7.6335, 9.8107) centre (-7.2678, 10.0033) ccw
  arc A520 (-7.47, 9.4583) -> (-7.6335, 9.8107) centre (-11.0364, 8.0181) ccw
  arc A521 (-7.5431, 9.1716) -> (-7.47, 9.4583) centre (-7.7019, 9.3647) ccw
  arc A522 (-7.5431, 9.1716) -> (-7.5957, 9.128) centre (0, 0) ccw
  arc A523 (-7.891, 9.11) -> (-7.5957, 9.128) centre (-7.7556, 9.3202) ccw
  arc A524 (-8.2065, 9.3366) -> (-7.891, 9.11) centre (-5.8081, 12.3433) ccw
  arc A525 (-8.2065, 9.3366) -> (-8.2664, 9.3764) centre (-8.4642, 9.0135) ccw
  arc A526 (-8.2664, 9.3764) -> (-8.7311, 9.5938) centre (-10.2609, 5.7181) ccw
  arc A527 (-8.7311, 9.5938) -> (-8.7832, 9.5841) centre (-8.7494, 9.5473) ccw
  arc A528 (-8.7832, 9.5841) -> (-9.0137, 9.3677) centre (0, 0) ccw
  arc A529 (-9.0137, 9.3677) -> (-9.0266, 9.3162) centre (-8.979, 9.3316) ccw
  arc A530 (-9.0266, 9.3162) -> (-8.8388, 8.8388) centre (-5.0626, 10.5997) ccw
  arc A531 (-8.8388, 8.8388) -> (-8.8029, 8.7766) centre (-8.4642, 9.0135) ccw
  arc A532 (-8.5966, 8.4475) -> (-8.8029, 8.7766) centre (-11.9543, 6.5717) ccw
  arc A533 (-8.6331, 8.1539) -> (-8.5966, 8.4475) centre (-8.8148, 8.3255) ccw
  arc A534 (-8.6331, 8.1539) -> (-8.6799, 8.1041) centre (0, 0) ccw
  arc A535 (-8.9706, 8.0492) -> (-8.6799, 8.1041) centre (-8.8626, 8.2747) ccw
  arc A536 (-9.312, 8.2344) -> (-8.9706, 8.0492) centre (-7.3093, 11.5181) ccw
  arc A537 (-9.312, 8.2344) -> (-9.3764, 8.2664) centre (-9.5272, 7.8816) ccw
  arc A538 (-9.3764, 8.2664) -> (-9.8646, 8.4238) centre (-10.8967, 4.387) ccw
  arc A539 (-9.8646, 8.4238) -> (-9.9152, 8.4077) centre (-9.877, 8.3754) ccw
  arc A540 (-9.9152, 8.4077) -> (-10.1167, 8.1641) centre (0, 0) ccw
  arc A541 (-10.1167, 8.1641) -> (-10.1231, 8.1114) centre (-10.0778, 8.1327) ccw
  arc A542 (-10.1231, 8.1114) -> (-9.8769, 7.6613) centre (-6.3511, 9.8817) ccw
  arc A543 (-9.8769, 7.6613) -> (-9.8335, 7.6041) centre (-9.5272, 7.8816) ccw
  arc A544 (-9.5875, 7.3034) -> (-9.8335, 7.6041) centre (-12.6837, 5.0216) ccw
  arc A545 (-9.587, 7.0076) -> (-9.5875, 7.3034) centre (-9.7888, 7.1551) ccw
  arc A546 (-9.587, 7.0076) -> (-9.6271, 6.9523) centre (0, 0) ccw
  arc A547 (-9.9087, 6.8614) -> (-9.6271, 6.9523) centre (-9.8298, 7.0986) ccw
  arc A548 (-10.2706, 7.0024) -> (-9.9087, 6.8614) centre (-8.6953, 10.5111) ccw
  arc A549 (-10.2706, 7.0024) -> (-10.3385, 7.026) centre (-10.4399, 6.6254) ccw
  arc A550 (-10.3385, 7.026) -> (-10.8426, 7.121) centre (-11.3606, 2.9867) ccw
  arc A551 (-10.8426, 7.121) -> (-10.8907, 7.0987) centre (-10.8488, 7.0714) ccw
  arc A552 (-10.8907, 7.0987) -> (-11.0602, 6.8317) centre (0, 0) ccw
  arc A553 (-11.0602, 6.8317) -> (-11.0599, 6.7787) centre (-11.0176, 6.8055) ccw
  arc A554 (-11.0599, 6.7787) -> (-10.7593, 6.363) centre (-7.5396, 9.0077) ccw
  arc A555 (-10.7593, 6.363) -> (-10.709, 6.3116) centre (-10.4399, 6.6254) ccw
  arc A556 (-10.4273, 6.0442) -> (-10.709, 6.3116) centre (-13.213, 3.3923) ccw